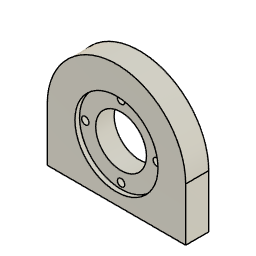
KS5N-IG36P_Mount1 (Autodesk Fusion 360 design; units mm, degrees)
Autodesk Fusion 360 part; units mm, degrees
note: some values were not read from the file. Chosen so that the rebuilt part matches the saved one: a direction; which face or edge a step refers to. Set by a fixed rule: which sketch regions a step uses.
sketch "スケッチ1" plane through (0, 0, 0) normal (0, 0, 1) x (1, 0, 0)
  line L0 (30, 5) -> (-30, 5)
  line L1 (-30, 5) -> (-30, -5)
  line L2 (-30, -5) -> (30, -5)
  line L3 (30, -5) -> (30, 5)
  line L4 (30, 5) -> (-30, -5) construction
  line L5 (-30, 5) -> (30, -5) construction
  dimension "d1" = 60
  dimension "d2" = 10
  constraint horizontal L0
  constraint perpendicular L0 L1
  constraint parallel L0 L2
  constraint parallel L1 L3
  constraint coincident L4 origin
  constraint coincident L5 origin
  measures "d1" distance of L1.end L2.end
  measures "d2" distance of L0.end L1.end
extrude "押し出し1" add sketch "スケッチ1" along normal blind 55
sketch "スケッチ2" plane through (0, -5, 0) normal (0, -1, 0) x (1, 0, 0)
  line L0 (-30, 0) -> (30, 0)
  line L1 (30, 0) -> (30, 55)
  line L2 (30, 55) -> (-30, 55)
  line L3 (-30, 55) -> (-30, 0)
  line L4 (0, 0) -> (0, 25)
  circle A0 centre (0, 25) radius 11
  circle A1 centre (0, 25) radius 18
  dimension "d5" = 25
  dimension "d6" = 22
  dimension "d7" = 36
  constraint coincident L4.start origin
  constraint perpendicular L0 L4
  constraint coincident L4.end A0.centre
  constraint concentric A0 A1
  measures "d5" distance of L4.start L4.end
  measures "d6" diameter of A0
  measures "d7" diameter of A1
extrude "押し出し2" cut sketch "スケッチ2" against normal blind 10 contours A0
extrude "押し出し3" cut sketch "スケッチ2" against normal blind 2 contours A1
sketch "スケッチ3" plane through (0, 0, 0) normal (0, 0, -1) x (1, 0, 0)
  line L0 (30, -5) -> (30, 5)
  line L1 (30, 5) -> (-30, 5)
  line L2 (-30, 5) -> (-30, -5)
  line L3 (-30, -5) -> (30, -5)
  line L4 (0, 0) -> (15, 0)
  line L5 (0, 0) -> (-15, 0)
  circle A0 centre (-15, 0) radius 2
  circle A1 centre (15, 0) radius 2
  dimension "d12" = 15
  dimension "d13" = 15
  dimension "d14" = 4
  dimension "d15" = 4
  constraint coincident L4.start L5.start
  constraint parallel L3 L4
  constraint parallel L4 L5
  constraint coincident L5.end A0.centre
  constraint coincident L4.end A1.centre
  measures "d12" distance of L4.start L4.end
  measures "d13" distance of L4.start L5.end
  measures "d14" diameter of A0
  measures "d15" diameter of A1
extrude "押し出し4" cut sketch "スケッチ3" against normal blind 10 contours A0 | A1
fillet "フィレット1" radius 30 2 edges at (-30, 0, 55) (30, 0, 55)
sketch "スケッチ4" plane through (0, -3, 0) normal (0, -1, 0) x (1, 0, 0)
  circle A0 centre (0, 25) radius 11
  circle A1 centre (0, 25) radius 18
  line L0 (0, 25) -> (-18, 25)
  line L1 (0, 25) -> (0, 43)
  line L2 (0, 25) -> (18, 25)
  line L3 (0, 25) -> (0, 7)
  line L4 (-11, 25) -> (-18, 25)
  line L5 (0, 36) -> (0, 43)
  line L6 (11, 25) -> (18, 25)
  line L7 (0, 14) -> (0, 7)
  circle A2 centre (-14.5, 25) radius 1.5
  circle A3 centre (0, 39.5) radius 1.5
  circle A4 centre (14.5, 25) radius 1.5
  circle A5 centre (0, 10.5) radius 1.5
  dimension "d22" = 3
  dimension "d23" = 3
  dimension "d24" = 3
  dimension "d25" = 3
  constraint coincident A0.centre A1.centre
  constraint coincident A1 L0.end
  constraint horizontal L0
  constraint coincident A1 L1.end
  constraint perpendicular L0 L1
  constraint coincident A1 L2.end
  constraint perpendicular L1 L2
  constraint coincident A1 L3.end
  constraint perpendicular L0 L3
  constraint coincident L0 L4.start
  constraint coincident A0 L4.start
  constraint coincident A0 L5.start
  constraint coincident L1 L5.start
  constraint coincident A0 L6.start
  constraint coincident L2 L6.start
  constraint coincident A0 L7.start
  constraint parallel L3 L7
  constraint midpoint L4 A2.centre
  constraint midpoint L5 A3.centre
  constraint midpoint L6 A4.centre
  constraint midpoint L7 A5.centre
  measures "d22" diameter of A2
  measures "d23" diameter of A3
  measures "d24" diameter of A4
  measures "d25" diameter of A5
extrude "押し出し5" cut sketch "スケッチ4" against normal blind 8 contours L2 L6 A4 | L2 L6 A4 | L1 L5 A3 | L1 L5 A3 | L3 L7 A5 | L3 L7 A5 | L0 L4 A2 | L0 L4 A2
extrude "押し出し6" cut 1 faces at (25.6667, 0, 0) along direction (0, 0, 1) blind 2
sketch "スケッチ5" plane through (0, -3, 0) normal (0, -1, 0) x (1, 0, 0)
  circle A0 centre (0, 39.5) radius 1.5
  circle A1 centre (0, 10.5) radius 1.5
  circle A2 centre (-14.5, 25) radius 1.5
  circle A3 centre (14.5, 25) radius 1.5
  circle A4 centre (0, 25) radius 11
  circle A5 centre (0, 25) radius 18
  circle A6 centre (0, 39.5) radius 1.6
  circle A7 centre (-14.5, 25) radius 1.6
  circle A8 centre (14.5, 25) radius 1.6
  circle A9 centre (0, 10.5) radius 1.6
  dimension "d38" = 3.2
  dimension "d39" = 3.2
  dimension "d40" = 3.2
  dimension "d41" = 3.2
  constraint concentric A0 A6
  constraint concentric A2 A7
  constraint concentric A3 A8
  constraint concentric A1 A9
  measures "d38" diameter of A6
  measures "d39" diameter of A7
  measures "d40" diameter of A8
  measures "d41" diameter of A9
extrude "押し出し7" cut sketch "スケッチ5" against normal blind 14 contours A6 | A7 | A8 | A9
sketch "スケッチ6" plane through (0, 0, 10) normal (0, 0, -1) x (1, 0, 0)
  circle A0 centre (15, 0) radius 2
  circle A1 centre (15, 0) radius 1.25
  dimension "d44" = 2.5
  constraint concentric A0 A1
  measures "d44" diameter of A1
extrude "押し出し8" add sketch "スケッチ6" along normal blind 8
sketch "スケッチ7" plane through (0, 0, 10) normal (0, 0, -1) x (1, 0, 0)
  circle A0 centre (-15, 0) radius 2
  circle A1 centre (-15, 0) radius 1.25
  dimension "d47" = 2.5
  constraint concentric A0 A1
  measures "d47" diameter of A1
extrude "押し出し9" add sketch "スケッチ7" along normal blind 8
sketch "スケッチ8" plane through (0, -3, 0) normal (0, -1, 0) x (1, 0, 0)
  circle A0 centre (0, 39.5) radius 1.6
  circle A1 centre (14.5, 25) radius 1.6
  circle A2 centre (-14.5, 25) radius 1.6
  circle A3 centre (0, 10.5) radius 1.6
  circle A4 centre (0, 25) radius 11
  circle A5 centre (0, 25) radius 18
  circle A6 centre (0, 25) radius 15.5
  line L0 (0, 25) -> (0, 40.5)
  line L1 (0, 25) -> (0, 9.5)
  line L2 (0, 25) -> (15.5, 25)
  line L3 (0, 25) -> (-15.5, 25)
  circle A7 centre (0, 40.5) radius 1.6
  circle A8 centre (0, 9.5) radius 1.6
  circle A9 centre (-15.5, 25) radius 1.6
  circle A10 centre (15.5, 25) radius 1.6
  dimension "d50" = 31
  dimension "d51" = 3.2
  dimension "d52" = 3.2
  dimension "d53" = 3.2
  dimension "d54" = 3.2
  constraint concentric A4 A6
  constraint coincident A4.centre A5.centre
  constraint coincident A6 L0.end
  constraint vertical L0
  constraint coincident A6 L1.end
  constraint parallel L0 L1
  constraint coincident A6 L2.end
  constraint perpendicular L1 L2
  constraint coincident A6 L3.end
  constraint parallel L2 L3
  constraint coincident L0.end A7.centre
  constraint coincident L1.end A8.centre
  constraint coincident L3.end A9.centre
  constraint coincident L2.end A10.centre
  measures "d50" diameter of A6
  measures "d51" diameter of A7
  measures "d52" diameter of A8
  measures "d53" diameter of A9
  measures "d54" diameter of A10
extrude "押し出し10" cut sketch "スケッチ8" against normal blind 8 contours A0 A6 A7 | A1 A6 A10 | A2 A6 A9 | A3 A6 A8 picked at (0.2414, 41.7429) picked at (16.7609, 25.0784) picked at (-16.7365, 24.7281) picked at (0.2414, 8.2571)
extrude "押し出し11" add sketch "スケッチ8" against normal blind 8 contours A0 L0 A7 | A0 L0 A7 | A1 L2 A10 | A1 L2 A10 | A2 L3 A9 | A2 L3 A9 | A3 L1 A8 | A3 L1 A8
extrude "押し出し12" cut sketch "スケッチ8" against normal blind 8 contours A0 A6 A7 | A0 A6 A7 | A0 A6 A7 | A1 A6 A10 | A1 A6 A10 | A2 A6 A9 | A1 A6 A10 | A2 A6 A9 | A3 A6 A8 | A3 A6 A8 | A3 A6 A8 picked at (-15.3365, 26.4873) picked at (-15.3365, 23.5127)
